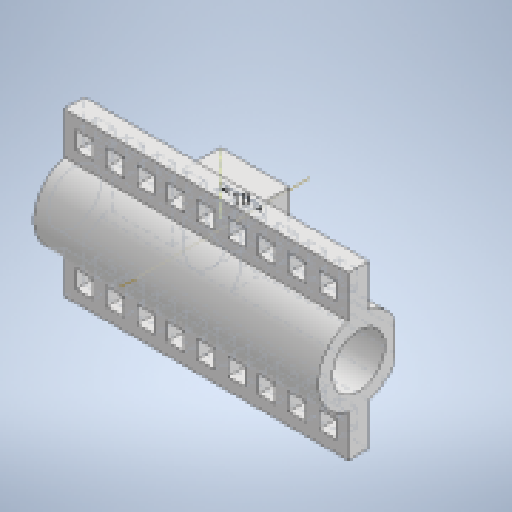
# Autodesk Inventor part: carriage
Saved by Autodesk Inventor 2023 (Build 270158000, 158)
## iProperties
Created: 2022-09-28
Part Number: carriage
Material: Generic
Document SubType Name: Modeling
Designer: carso
Density: 1 g/cm^3
Appearance: Default
Author: carso
Autodesk Inventor part; units mm, degrees
ref_plane "YZ Plane" through (0, 0, 0) normal (1, 0, 0) x (0, 1, 0)
ref_plane "XZ Plane" through (0, 0, 0) normal (0, 1, 0) x (-1, 0, 0)
ref_plane "XY Plane" through (0, 0, 0) normal (0, 0, 1) x (1, 0, 0)
sketch "Sketch1" plane through (0, 0, 0) normal (1, 0, 0) x (0, 1, 0)
  circle A0 centre (0, 0) radius 6.5
  circle A1 centre (0, 0) radius 10
  line L0 (-20, 2.5) -> (20, 2.5)
  line L1 (20, 2.5) -> (20, -2.5)
  line L2 (20, -2.5) -> (-20, -2.5)
  line L3 (-20, -2.5) -> (-20, 2.5)
  line L4 (-20, 2.5) -> (20, -2.5) construction
  line L5 (20, 2.5) -> (-20, -2.5) construction
  line L6 (7.5, 9) -> (7.5, -9)
  line L7 (7.5, -9) -> (-7.5, -9)
  line L8 (-7.5, -9) -> (-7.5, 9)
  line L9 (-7.5, 9) -> (7.5, 9)
  line L10 (7.5, 9) -> (-7.5, -9) construction
  line L11 (7.5, -9) -> (-7.5, 9) construction
  point P0 (-9.6825, -2.5)
  point P1 (-9.6825, 2.5)
  point P2 (9.6825, 2.5)
  point P3 (9.6825, -2.5)
  point P4 (-7.5, -6.6144)
  point P5 (-4.3589, -9)
  point P6 (7.5, -6.6144)
  point P7 (4.3589, -9)
  point P8 (-7.5, 6.6144)
  point P9 (7.5, 6.6144)
  point P10 (4.3589, 9)
  point P11 (-4.3589, 9)
  dimension "d3" = 13
  dimension "d4" = 3.5
  dimension "d7" = 40
  dimension "d8" = 5
  dimension "d27" = 15
  dimension "d28" = 2.5
  constraints: 24 end point, 4 midpoint, 4 parallel, 2 centre point, 2 coincident, 2 perpendicular, 1 horizontal, 1 vertical
  measures "d3" diameter of A0
  measures "d4" radial gap between concentric circles of A1 A0
  measures "d7" distance of L0.start L0.end
  measures "d8" distance of L0.end L1.end
  measures "d27" distance of L6.end L7.end
  measures "d28" distance edge to line of A0 L7
extrude "Extrusion2" add sketch "Sketch1" along normal blind 70 contours A0 L0 L6 L2 | A0 L0 L8 A1 L9 L6 | L2 L6 A1 L7 L8 A0 | A0 L2 L8 L0 | L6 A1 L0 | L0 A1 L2 L6 | L2 A1 L6 | L8 L2 A1 L0 | L0 A1 L8 | L0 L1 L2 A1 | L8 A1 L2 | L6 L7 A1 | A1 L2 L3 L0 | L9 A1 | A1 L7 L8
sketch "Sketch3" plane through (0, -20, -2.5) normal (0, 0, -1) x (-1, 0, 0)
  line L0 (-67, 3) -> (-62.6825, 3)
  line L1 (-62.6825, 3) -> (-62.6825, 7.3175)
  line L2 (-62.6825, 7.3175) -> (-67, 7.3175)
  line L3 (-67, 7.3175) -> (-67, 3)
  line L4 (0, 0) -> (-70, 0) projected
  line L5 (0, 10.3175) -> (-70, 10.3175) projected
  line L6 (-70, 0) -> (-70, 10.3175) projected
  line L7 (-59.5318, 7.3175) -> (-59.5318, 3)
  line L8 (-59.5318, 3) -> (-55.2143, 3)
  line L9 (-55.2143, 3) -> (-55.2143, 7.3175)
  line L10 (-55.2143, 7.3175) -> (-59.5318, 7.3175)
  line L11 (-52.0636, 7.3175) -> (-52.0636, 3)
  line L12 (-52.0636, 3) -> (-47.7461, 3)
  line L13 (-47.7461, 3) -> (-47.7461, 7.3175)
  line L14 (-47.7461, 7.3175) -> (-52.0636, 7.3175)
  line L15 (-44.5954, 7.3175) -> (-44.5954, 3)
  line L16 (-44.5954, 3) -> (-40.2779, 3)
  line L17 (-40.2779, 3) -> (-40.2779, 7.3175)
  line L18 (-40.2779, 7.3175) -> (-44.5954, 7.3175)
  line L19 (-37.1272, 7.3175) -> (-37.1272, 3)
  line L20 (-37.1272, 3) -> (-32.8097, 3)
  line L21 (-32.8097, 3) -> (-32.8097, 7.3175)
  line L22 (-32.8097, 7.3175) -> (-37.1272, 7.3175)
  line L23 (-29.659, 7.3175) -> (-29.659, 3)
  line L24 (-29.659, 3) -> (-25.3415, 3)
  line L25 (-25.3415, 3) -> (-25.3415, 7.3175)
  line L26 (-25.3415, 7.3175) -> (-29.659, 7.3175)
  line L27 (-22.1908, 7.3175) -> (-22.1908, 3)
  line L28 (-22.1908, 3) -> (-17.8733, 3)
  line L29 (-17.8733, 3) -> (-17.8733, 7.3175)
  line L30 (-17.8733, 7.3175) -> (-22.1908, 7.3175)
  line L31 (-14.7226, 7.3175) -> (-14.7226, 3)
  line L32 (-14.7226, 3) -> (-10.4051, 3)
  line L33 (-10.4051, 3) -> (-10.4051, 7.3175)
  line L34 (-10.4051, 7.3175) -> (-14.7226, 7.3175)
  line L35 (-7.2544, 7.3175) -> (-7.2544, 3)
  line L36 (-7.2544, 3) -> (-2.9369, 3)
  line L37 (-2.9369, 3) -> (-2.9369, 7.3175)
  line L38 (-2.9369, 7.3175) -> (-7.2544, 7.3175)
  line L39 (-67, 36.9995) -> (-67, 32.682)
  line L40 (-67, 32.682) -> (-62.6825, 32.682)
  line L41 (-62.6825, 32.682) -> (-62.6825, 36.9995)
  line L42 (-62.6825, 36.9995) -> (-67, 36.9995)
  line L43 (-59.5318, 36.9995) -> (-59.5318, 32.682)
  line L44 (-59.5318, 32.682) -> (-55.2143, 32.682)
  line L45 (-55.2143, 32.682) -> (-55.2143, 36.9995)
  line L46 (-55.2143, 36.9995) -> (-59.5318, 36.9995)
  line L47 (-52.0636, 36.9995) -> (-52.0636, 32.682)
  line L48 (-52.0636, 32.682) -> (-47.7461, 32.682)
  line L49 (-47.7461, 32.682) -> (-47.7461, 36.9995)
  line L50 (-47.7461, 36.9995) -> (-52.0636, 36.9995)
  line L51 (-44.5954, 36.9995) -> (-44.5954, 32.682)
  line L52 (-44.5954, 32.682) -> (-40.2779, 32.682)
  line L53 (-40.2779, 32.682) -> (-40.2779, 36.9995)
  line L54 (-40.2779, 36.9995) -> (-44.5954, 36.9995)
  line L55 (-37.1272, 36.9995) -> (-37.1272, 32.682)
  line L56 (-37.1272, 32.682) -> (-32.8097, 32.682)
  line L57 (-32.8097, 32.682) -> (-32.8097, 36.9995)
  line L58 (-32.8097, 36.9995) -> (-37.1272, 36.9995)
  line L59 (-29.659, 36.9995) -> (-29.659, 32.682)
  line L60 (-29.659, 32.682) -> (-25.3415, 32.682)
  line L61 (-25.3415, 32.682) -> (-25.3415, 36.9995)
  line L62 (-25.3415, 36.9995) -> (-29.659, 36.9995)
  line L63 (-22.1908, 36.9995) -> (-22.1908, 32.682)
  line L64 (-22.1908, 32.682) -> (-17.8733, 32.682)
  line L65 (-17.8733, 32.682) -> (-17.8733, 36.9995)
  line L66 (-17.8733, 36.9995) -> (-22.1908, 36.9995)
  line L67 (-14.7226, 36.9995) -> (-14.7226, 32.682)
  line L68 (-14.7226, 32.682) -> (-10.4051, 32.682)
  line L69 (-10.4051, 32.682) -> (-10.4051, 36.9995)
  line L70 (-10.4051, 36.9995) -> (-14.7226, 36.9995)
  line L71 (-7.2544, 36.9995) -> (-7.2544, 32.682)
  line L72 (-7.2544, 32.682) -> (-2.9369, 32.682)
  line L73 (-2.9369, 32.682) -> (-2.9369, 36.9995)
  line L74 (-2.9369, 36.9995) -> (-7.2544, 36.9995)
  line L75 (0, 0) -> (0, 10.3175) projected
  line L76 (0, 40) -> (-70, 40) projected
  line L77 (0, 29.6825) -> (-70, 29.6825) projected
  point P0 (0, 20)
  point P1 (-64.8412, 7.3175)
  point P2 (-57.373, 7.3175)
  point P3 (-49.9048, 7.3175)
  point P4 (-42.4366, 7.3175)
  point P5 (-34.9684, 7.3175)
  point P6 (-27.5002, 7.3175)
  point P7 (-20.032, 7.3175)
  point P8 (-12.5638, 7.3175)
  point P9 (-5.0956, 7.3175)
  point P10 (-64.8412, 36.9995)
  point P11 (-57.373, 36.9995)
  point P12 (-49.9048, 36.9995)
  point P13 (-42.4366, 36.9995)
  point P14 (-34.9684, 36.9995)
  point P15 (-27.5002, 36.9995)
  point P16 (-20.032, 36.9995)
  point P17 (-12.5638, 36.9995)
  point P18 (-5.0956, 36.9995)
  point P19 (0, 5.1588)
  dimension "d9" = 3
  dimension "d10" = 3
  dimension "d11" = 3
  dimension "d12" = 4.3175
  dimension "d13" = 4.3175
  dimension "d16" = 7.4682
  dimension "d19" = 29.682
  dimension "d22" = 2.9369
  dimension "d23" = 3.0005
  dimension "d24" = 2.9995
  constraints: 144 end point, 2 collinear, 2 horizontal, 2 midpoint, 2 parallel, 1 perpendicular, 1 vertical, 151 other
  measures "d9" distance between parallel lines of L4 L0
  measures "d10" distance between parallel lines of L5 L2
  measures "d11" distance between parallel lines of L6 L3
  measures "d12" distance from line of point (-64.841, 7.318) L0
  measures "d13" distance between parallel lines of L3 L1
  measures "d16" distance of L2.end L7.start
  measures "d19" distance of L2.end L39.start
  measures "d22" distance from line of point (0, 5.159) L37
  measures "d23" distance between parallel lines of L76 L42
  measures "d24" distance between parallel lines of L77 L40
extrude "Extrusion3" cut sketch "Sketch3" against normal blind 5 contours L3 L2 L1 L0 | L10 L9 L8 L7 | L14 L13 L12 L11 | L18 L17 L16 L15 | L22 L21 L20 L19 | L26 L25 L24 L23 | L30 L29 L28 L27 | L34 L33 L32 L31 | L38 L37 L36 L35 | L42 L41 L40 L39 | L46 L45 L44 L43 | L50 L49 L48 L47 | L54 L53 L52 L51 | L58 L57 L56 L55 | L62 L61 L60 L59 | L66 L65 L64 L63 | L70 L69 L68 L67 | L74 L73 L72 L71
sketch "Sketch4" plane through (0, -7.5, -9) normal (0, -1, 0) x (1, 0, 0)
  line L0 (0, 2.3856) -> (0, 0) projected
  line L1 (0, 0) -> (15, 0)
  line L2 (15, 0) -> (15, -12)
  line L3 (15, -12) -> (0, -12)
  line L4 (0, -12) -> (0, 0)
  line L5 (0, 0) -> (70, 0) projected
  line L6 (15, -12) -> (32, -12)
  line L7 (32, -12) -> (32, 0)
  line L8 (32, 0) -> (15, 0)
  line L9 (15, 0) -> (15, -12)
  point P0 (0, 9)
  dimension "d29" = 15
  dimension "d30" = 12
  dimension "d31" = 17
  constraints: 16 end point, 4 parallel, 2 horizontal, 2 perpendicular, 1 point on line
  measures "d29" distance of L2.end L3.end
  measures "d30" distance between parallel lines of L1 L3
  measures "d31" distance of L8.end L7.end
extrude "Extrusion4" add sketch "Sketch4" against normal blind 15 contours L5 L7 L6 L2
sketch "Sketch5" plane through (32, -7.5, -21) normal (0, 0, -1) x (-1, 0, 0)
  line L0 (17, 0) -> (17, 15) projected
  line L1 (17, 7.5) -> (7, 7.5)
  point P0 (32, 7.5)
  dimension "d34" = 10
  constraints: 2 end point, 1 horizontal, 1 midpoint
  measures "d34" distance of L1.start L1.end
hole "Hole1" at (25, 0, -2.5) direction (0, 0, -1) diameter 3 depth 20 counterbore diameter 10 counterbore depth 10
fillet "Fillet1" radius 6 2 edges at (51, -7.5, -9) (51, 7.5, -9)
equation "\"d13\" = d12"
body "Solid2"
